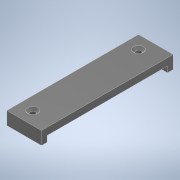
# Autodesk Inventor part: Holder V1
Saved by Autodesk Inventor 2022 (Build 260153000, 153)
## iProperties
Created: 2022-04-15
Part Number: Holder V1
Material: Acetal Resin, Black
Document SubType Name: Modeling
Designer: Caleb
Density: 1.425 g/cm^3
Appearance: Smooth - Black
Author: Caleb
Autodesk Inventor part; units mm, degrees
ref_plane "YZ Plane" through (0, 0, 0) normal (1, 0, 0) x (0, 1, 0)
ref_plane "XZ Plane" through (0, 0, 0) normal (0, 1, 0) x (-1, 0, 0)
ref_plane "XY Plane" through (0, 0, 0) normal (0, 0, 1) x (1, 0, 0)
sketch "Sketch1" plane through (0, 0, 0) normal (0, 1, 0) x (-1, 0, 0)
  line L0 (-6.35, -24.13) -> (6.35, -24.13)
  line L1 (6.35, -24.13) -> (6.35, 24.13)
  line L2 (6.35, 24.13) -> (-6.35, 24.13)
  line L3 (-6.35, 24.13) -> (-6.35, -24.13)
  line L4 (-6.35, -24.13) -> (6.35, 24.13) construction
  line L5 (6.35, -24.13) -> (-6.35, 24.13) construction
  point P0 (0, 0)
  dimension "d0" = 12.7
  dimension "d1" = 48.26
  constraints: 12 end point, 2 midpoint, 2 parallel, 1 horizontal, 1 perpendicular
  measures "d0" distance of L2.end L1.end
  measures "d1" distance of L1.end L0.end
extrude "Extrusion1" add sketch "Sketch1" along normal blind 4.7625
sketch "Sketch2" plane through (6.35, 0, 24.13) normal (1, 0, 0) x (0, 0, -1)
  line L0 (48.26, 0) -> (0, 0) projected
  line L1 (2.08, 0) -> (46.18, 0)
  line L2 (46.18, 0) -> (46.18, 2.15)
  line L3 (46.18, 2.15) -> (2.08, 2.15)
  line L4 (2.08, 2.15) -> (2.08, 0)
  line L5 (24.13, 3.9864) -> (24.13, -0.9105)
  point P0 (24.13, 0)
  dimension "d4" = 2.15
  dimension "d5" = 44.1
  constraints: 10 end point, 2 parallel, 1 horizontal, 1 perpendicular, 1 point on line, 1 vertical, 1 other
  measures "d4" distance of L3.end L1.start
  measures "d5" distance of L2.end L3.end
extrude "Extrusion2" cut sketch "Sketch2" against normal blind 3.175
sketch "Sketch3" plane through (0, 4.7625, 0) normal (0, 1, 0) x (1, 0, 0)
  line L0 (-5.9119, 0) -> (5.9776, 0)
  line L1 (-6.35, 24.13) -> (-6.35, -24.13) projected
  line L2 (-6.35, -24.13) -> (6.35, -24.13) projected
  point P0 (0, 0)
  point P1 (-1.5875, -19.3675)
  point P2 (-1.5875, 19.3675)
  dimension "d18" = 4.7625
  dimension "d19" = 4.7625
  constraints: 2 end point, 1 horizontal, 1 point on line, 1 symmetric about line
  measures "d18" distance from line of L1 point (-1.587, -19.367)
  measures "d19" distance from line of L2 point (-1.587, -19.367)
hole "Hole1" at (-1.5875, 4.7625, 19.3675) at (-1.5875, 4.7625, -19.3675) direction (0, -1, 0) diameter 2.0574 end through all countersink diameter 3.7084 countersink angle 82 clearance for "Flat Head Machine Screw (82)" size "#1" standard "Ansi Unified Screw Threads"
equation "\"d19\" = d18"
body "Solid1"
